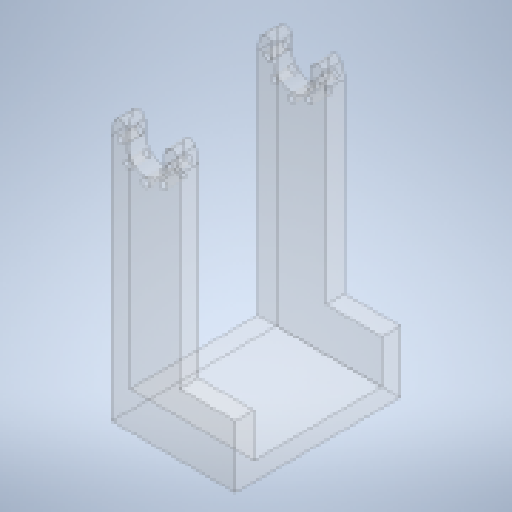
# Autodesk Inventor part: 부품56
Saved by Autodesk Inventor 2024 (Build 280153000, 153)
## iProperties
Created: 2024-09-07
Part Number: 부품56
Material: PMMA 플라스틱
Document SubType Name: Modeling
Designer: Eungang
Density: 1.188 g/cm^3
Appearance: 폴리카보네이트 - 선명
Mass: 41.4666 g
Surface Area: 152.736 cm^2
Volume: 34.9046 cm^3
Author: Eungang
Autodesk Inventor part; units mm, degrees
ref_plane "YZ Plane" through (0, 0, 0) normal (1, 0, 0) x (0, 1, 0)
ref_plane "XZ Plane" through (0, 0, 0) normal (0, 1, 0) x (-1, 0, 0)
ref_plane "XY Plane" through (0, 0, 0) normal (0, 0, 1) x (1, 0, 0)
sketch "스케치1" plane through (0, 0, 0) normal (0, 0, 1) x (1, 0, 0)
  circle A0 centre (0, 8) radius 1.05 projected
  line L0 (6.1695, 0) -> (-5.6569, 0)
  circle A1 centre (0, 0) radius 11 projected
  line L1 (11, -20) -> (31, -20) projected
  line L2 (11, 0) -> (11, -20) projected
  arc A2 (11, 0) -> (7.5778, 7.9735) centre (0, 0) ccw projected
  arc A3 (-7.5778, 7.9735) -> (-11, 0) centre (0, 0) ccw projected
  line L3 (-11, -40) -> (-11, 0) projected
  line L4 (31, -40) -> (-11, -40) projected
  line L5 (31, -20) -> (31, -40) projected
  circle A4 centre (5.6569, 5.6569) radius 1.2 projected
  circle A5 centre (-8, 0) radius 1.2 projected
  circle A6 centre (-5.6569, 5.6569) radius 1.2 projected
  circle A7 centre (-5.6569, -5.6569) radius 1.2 projected
  circle A8 centre (5.6569, -5.6569) radius 1.2 projected
  circle A9 centre (0, -8) radius 1.2 projected
  circle A10 centre (8, 0) radius 1.2 projected
  arc A11 (-10.0222, 4.5338) -> (10.0222, 4.5338) centre (0, 0) ccw
  arc A12 (-4.2, 0) -> (4.2, 0) centre (0, 0) ccw
  line L6 (4.2, 0) -> (-4.2, 0)
  line L7 (-4.2, 0) -> (-4.2, 6.5238)
  line L8 (-4.2, 13.5959) -> (4.2, 13.5959)
  line L9 (4.2, 6.5238) -> (4.2, 0)
  arc A13 (-7.5778, 7.9735) -> (7.5778, 7.9735) centre (0, 0) ccw
  arc A14 (7.5778, 7.9735) -> (4.2, 6.5238) centre (6.2, 6.5238) ccw
  arc A15 (-4.2, 6.5238) -> (-7.5778, 7.9735) centre (-6.2, 6.5238) ccw
  point P0 (-6.2, 0)
  point P1 (4.2, 10.1666)
  point P2 (-4.2, 10.1666)
  point P3 (-7.5778, 7.9735)
  point P4 (7.5778, 7.9735)
  dimension "d20" = 2
  constraints: 13 point on circle, 10 end point, 6 point on line, 5 centre point, 4 tangent, 2 coincident, 2 equal radius, 2 horizontal, 2 parallel, 1 perpendicular
  measures "d20" radius of A14
extrude "돌출1" add sketch "스케치1" along normal blind 6 contours L9 A14 A1 A15 L7 A12
sketch "스케치3" plane through (0, 0, 6) normal (0, 0, 1) x (1, 0, 0)
  line L0 (31, -40) -> (31, -20) projected
  line L1 (11, -20) -> (31, -20)
  line L2 (31, -20) -> (31, -40)
  line L3 (31, -40) -> (11, -40)
  line L4 (11, -40) -> (11, -20)
  arc A0 (-7.5778, 7.9735) -> (7.5778, 7.9735) centre (0, 0) ccw projected
  circle A1 centre (-8, 0) radius 1.2 projected
  circle A2 centre (-5.6569, -5.6569) radius 1.2 projected
  circle A3 centre (5.6569, -5.6569) radius 1.2 projected
  circle A4 centre (0, -8) radius 1.2 projected
  circle A5 centre (8, 0) radius 1.2 projected
  line L5 (11, -40) -> (-11, -40)
  line L6 (-11, -40) -> (-11, -80)
  line L7 (-11, -80) -> (11, -80)
  line L8 (11, -80) -> (11, -40)
  line L9 (-11, -80) -> (29, -80)
  line L10 (29, -80) -> (29, -60)
  line L11 (29, -60) -> (-11, -60)
  line L12 (-11, -60) -> (-11, -80)
  line L13 (-11, -40) -> (11, -40)
  line L14 (11, -40) -> (11, 0)
  line L15 (11, 0) -> (-11, 0)
  line L16 (-11, 0) -> (-11, -40)
  arc A6 (7.5778, 7.9735) -> (4.2, 6.5238) centre (6.2, 6.5238) ccw projected
  line L17 (4.2, 6.5238) -> (4.2, 0) projected
  arc A7 (-4.2, 0) -> (4.2, 0) centre (0, 0) ccw projected
  line L18 (-4.2, 0) -> (-4.2, 6.5238) projected
  arc A8 (-4.2, 6.5238) -> (-7.5778, 7.9735) centre (-6.2, 6.5238) ccw projected
  point P0 (11, -60)
  dimension "d4" = 40
  constraints: 32 end point, 8 parallel, 4 horizontal, 4 perpendicular, 1 point on circle
  measures "d4" distance of L6.end L5.end
extrude "돌출2" add sketch "스케치3" against normal blind 6 contours L5 L16 A0 L14 L4 | L8 L11 L6 L5 | L11 L10 L9 L8 | L8 L7 L6 L11
sketch "스케치4" plane through (0, 0, 0) normal (0, 0, -1) x (-1, 0, 0)
  line L0 (11, 0) -> (11, -80) projected
  line L1 (-29, -60) -> (-29, -80) projected
  line L2 (11, -80) -> (-29, -80)
  line L3 (-29, -80) -> (-29, -60)
  line L4 (-29, -60) -> (11, -60)
  line L5 (11, -60) -> (11, -80)
  line L6 (11, -80) -> (-29, -80)
  line L7 (-29, -80) -> (-29, -74)
  line L8 (-29, -74) -> (11, -74)
  line L9 (11, -74) -> (11, -80)
  point P0 (0, 0)
  dimension "d7" = 6
  constraints: 16 end point, 4 parallel, 2 horizontal, 2 perpendicular, 1 point on line
  measures "d7" distance of L6.end L7.end
extrude "돌출3" add sketch "스케치4" along normal blind 41.2 contours L0 L2 L1 L8
sketch "스케치5" plane through (0, 0, -41.2) normal (0, 0, -1) x (-1, 0, 0)
  circle A0 centre (0, 0) radius 11 projected
  circle A1 centre (5.6569, -5.6569) radius 1.15
  circle A2 centre (8, 0) radius 1.15
  circle A3 centre (5.6569, 5.6569) radius 1.15
  circle A4 centre (0, 8) radius 1.15
  circle A5 centre (-5.6569, 5.6569) radius 1.15
  circle A6 centre (-8, 0) radius 1.15
  circle A7 centre (-5.6569, -5.6569) radius 1.15
  circle A8 centre (0, -8) radius 1.15
  line L0 (-11, 0) -> (-11, -60) projected
  line L1 (11, 0) -> (11, -80) projected
  line L2 (-11, 0) -> (11, 0)
  line L3 (11, 0) -> (11, -80)
  line L4 (11, -80) -> (-11, -80)
  line L5 (-11, -80) -> (-11, 0)
  line L6 (-29, -80) -> (-29, -60) projected
  line L7 (-29, -80) -> (-11, -80)
  line L8 (-11, -80) -> (-11, -60)
  line L9 (-11, -60) -> (-29, -60)
  line L10 (-29, -60) -> (-29, -80)
  line L11 (6.2, 0) -> (-6.2, 0)
  line L12 (-6.2, 15) -> (6.2, 15)
  arc A9 (-10.0222, 4.5338) -> (10.0222, 4.5338) centre (0, 0) ccw
  arc A10 (11, 0) -> (7.5778, 7.9735) centre (0, 0) ccw projected
  line L13 (11, 0) -> (11, -80) projected
  line L14 (11, -80) -> (-29, -80) projected
  line L15 (-29, -80) -> (-29, -60) projected
  line L16 (-29, -60) -> (-11, -60) projected
  line L17 (-11, -60) -> (-11, 0) projected
  arc A11 (-7.5778, 7.9735) -> (-11, 0) centre (0, 0) ccw projected
  arc A12 (-4.2, 6.5238) -> (-7.5778, 7.9735) centre (-6.2, 6.5238) ccw projected
  line L18 (-4.2, 6.5238) -> (-4.2, 0) projected
  arc A13 (-4.2, 0) -> (4.2, 0) centre (0, 0) ccw projected
  line L19 (4.2, 0) -> (4.2, 6.5238) projected
  arc A14 (7.5778, 7.9735) -> (4.2, 6.5238) centre (6.2, 6.5238) ccw projected
  circle A15 centre (-8, 0) radius 1.2 projected
  circle A16 centre (0, -8) radius 1.2 projected
  circle A17 centre (-5.6569, -5.6569) radius 1.2 projected
  circle A18 centre (5.6569, -5.6569) radius 1.2 projected
  circle A19 centre (5.6569, 5.6569) radius 1.2 projected
  circle A20 centre (8, 0) radius 1.2 projected
  circle A21 centre (-5.6569, 5.6569) radius 1.2 projected
  circle A22 centre (5.6569, 5.6569) radius 1.1
  circle A23 centre (0, 8) radius 1.1
  circle A24 centre (-5.6569, 5.6569) radius 1.1
  circle A25 centre (-8, 0) radius 1.1
  circle A26 centre (-5.6569, -5.6569) radius 1.1
  circle A27 centre (0, -8) radius 1.1
  circle A28 centre (5.6569, -5.6569) radius 1.1
  circle A29 centre (8, 0) radius 1.1
  point P0 (0, 0)
  point P1 (6.2, 9.0863)
  point P2 (-6.2, 9.0863)
  point P3 (11, 0)
  point P4 (9.2, 0)
  point P5 (6.8, 0)
  point P6 (6.85, 0)
  point P7 (9.15, 0)
  point P8 (7.5778, 7.9735)
  point P9 (-7.5778, 7.9735)
  point P10 (6.9, 0)
  point P11 (9.1, 0)
  point P12 (-6.9, 0)
  point P13 (-9.1, 0)
  point P14 (-9.15, 0)
  point P15 (-6.85, 0)
  dimension "d13" = 360
  dimension "d21" = 2.2
  dimension "d24" = 360
  constraints: 20 end point, 17 centre point, 5 parallel, 4 point on circle, 3 horizontal, 2 coincident, 2 perpendicular, 2 point on line, 1 concentric, 34 other
  measures "d21" diameter of A22
extrude "돌출4" add sketch "스케치5" along normal blind 6 contours L2 A20 L19 A14 A0 | L1 L4 L5 L0 A0 | A0 L2 A15 A13 A20 | A0 A12 L18 L2 A15 | L2 A2 A20 | L5 L7 L6 L9 | A15 L2 A6 | L2 A6 A15 | L2 A29 A2 | L2 A25 A6 | A6 L2 A25 | A1 | A3 | A5 | A7 | A8 | A16 | A17 | A18 | A19 | A21 picked at (7.9538, 1.1747) picked at (6.8885, 0.1795)
